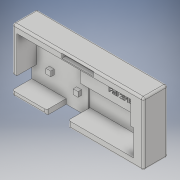
# Autodesk Inventor part: case3
Saved by Autodesk Inventor 2017 (Build 210142000, 142)
## iProperties
Created: 2016-12-02
Part Number: case3
Material: Generic
Document SubType Name: Modeling
Designer: SDL
Density: 1 g/cm^3
Appearance: Default
Author: SDL
Autodesk Inventor part; units mm, degrees
ref_plane "YZ Plane" through (0, 0, 0) normal (1, 0, 0) x (0, 1, 0)
ref_plane "XZ Plane" through (0, 0, 0) normal (0, 1, 0) x (-1, 0, 0)
ref_plane "XY Plane" through (0, 0, 0) normal (0, 0, 1) x (1, 0, 0)
sketch "Sketch1" plane through (0, 0, 0) normal (0, 0, 1) x (1, 0, 0)
  line L0 (0, 0) -> (133, 0)
  line L1 (133, 0) -> (133, 64)
  line L2 (133, 64) -> (0, 64)
  line L3 (0, 64) -> (0, 0)
  dimension "d0" = 133
  dimension "d1" = 64
  constraints: 8 end point, 2 parallel, 1 horizontal, 1 perpendicular
  measures "d0" distance of L2.end L1.end
  measures "d1" distance of L1.end L0.end
extrude "Extrusion1" add sketch "Sketch1" along normal blind 25
sketch "Sketch2" plane through (0, 0, 25) normal (0, 0, 1) x (1, 0, 0)
  line L0 (5, 5) -> (57, 5)
  line L1 (57, 5) -> (57, 57)
  line L2 (57, 57) -> (5, 57)
  line L3 (5, 57) -> (5, 5)
  dimension "d10" = 52
  dimension "d11" = 52
  constraints: 8 end point, 2 parallel, 1 horizontal, 1 perpendicular
  measures "d10" distance of L2.end L1.end
  measures "d11" distance of L1.end L0.end
extrude "Extrusion2" cut sketch "Sketch2" against normal blind 20
sketch "Sketch3" plane through (0, 0, 25) normal (0, 0, 1) x (1, 0, 0)
  line L0 (57, 57) -> (57, 5) projected
  line L1 (57, 7) -> (123, 7)
  line L2 (123, 7) -> (123, 33.5)
  line L3 (123, 33.5) -> (57, 33.5)
  line L4 (57, 33.5) -> (57, 7)
  point P0 (0, 0)
  dimension "d15" = 66
  dimension "d16" = 26.5
  constraints: 8 end point, 2 parallel, 1 horizontal, 1 perpendicular, 1 point on line
  measures "d15" distance of L3.end L2.end
  measures "d16" distance of L2.end L1.end
extrude "Extrusion3" cut sketch "Sketch3" against normal blind 22
sketch "Sketch4" plane through (0, 0, 3) normal (0, 0, 1) x (1, 0, 0)
  line L0 (123, 7) -> (57, 7) projected
  line L1 (57, 33.5) -> (123, 33.5) projected
  line L2 (123, 7) -> (110, 7)
  line L3 (110, 7) -> (110, 33.5)
  line L4 (110, 33.5) -> (123, 33.5)
  line L5 (123, 33.5) -> (123, 7)
  point P0 (0, 0)
  dimension "d19" = 13
  constraints: 8 end point, 2 parallel, 1 horizontal, 1 perpendicular, 1 point on line
  measures "d19" distance of L3.end L4.end
extrude "Extrusion4" cut sketch "Sketch4" against normal blind 25
sketch "Sketch5" plane through (0, 0, 25) normal (0, 0, 1) x (1, 0, 0)
  line L0 (57, 33.5) -> (110, 33.5) projected
  line L1 (57, 33.5) -> (120, 33.5)
  line L2 (120, 33.5) -> (120, 57)
  line L3 (120, 57) -> (57, 57)
  line L4 (57, 57) -> (57, 33.5)
  point P0 (0, 0)
  dimension "d22" = 63
  constraints: 8 end point, 2 parallel, 1 horizontal, 1 perpendicular
  measures "d22" distance of L3.end L2.end
extrude "Extrusion5" cut sketch "Sketch5" against normal blind 12
sketch "Sketch6" plane through (0, 0, 5) normal (0, 0, 1) x (1, 0, 0)
  line L0 (5.5, 56.5) -> (56, 5.5) construction
  line L1 (56, 55.5) -> (6, 5.5) construction
  line L2 (5.5, 56.5) -> (5.5, 53.5)
  line L3 (5.5, 53.5) -> (9.9, 53.5)
  line L4 (6, 5.5) -> (6, 22.2)
  line L5 (6, 22.2) -> (20.3, 22.2)
  line L6 (56, 5.5) -> (56, 18)
  line L7 (56, 18) -> (47.9, 18)
  line L8 (7.4, 56) -> (12.4, 56)
  line L9 (12.4, 56) -> (12.4, 51)
  line L10 (12.4, 51) -> (7.4, 51)
  line L11 (7.4, 51) -> (7.4, 56)
  line L12 (7.4, 56) -> (12.4, 51) construction
  line L13 (12.4, 56) -> (7.4, 51) construction
  line L14 (17.8, 24.7) -> (22.8, 24.7)
  line L15 (22.8, 24.7) -> (22.8, 19.7)
  line L16 (22.8, 19.7) -> (17.8, 19.7)
  line L17 (17.8, 19.7) -> (17.8, 24.7)
  line L18 (17.8, 24.7) -> (22.8, 19.7) construction
  line L19 (22.8, 24.7) -> (17.8, 19.7) construction
  line L20 (45.4, 20.5) -> (50.4, 20.5)
  line L21 (50.4, 20.5) -> (50.4, 15.5)
  line L22 (50.4, 15.5) -> (45.4, 15.5)
  line L23 (45.4, 15.5) -> (45.4, 20.5)
  line L24 (45.4, 20.5) -> (50.4, 15.5) construction
  line L25 (50.4, 20.5) -> (45.4, 15.5) construction
  point P0 (0, 0)
  point P1 (31.1232, 30.6232)
  dimension "d25" = 50
  dimension "d26" = 50
  dimension "d27" = 3
  dimension "d28" = 4.4
  dimension "d29" = 16.7
  dimension "d30" = 14.3
  dimension "d31" = 12.5
  dimension "d32" = 8.1
  dimension "d33" = 5
  dimension "d34" = 5
  dimension "d35" = 5
  dimension "d36" = 5
  dimension "d37" = 5
  dimension "d38" = 5
  constraints: 52 end point, 6 midpoint, 6 parallel, 6 perpendicular, 3 horizontal, 2 point on line
  measures "d25" distance of L0.end L1.end
  measures "d26" distance of L1.start L0.end
  measures "d27" distance of L0.start L2.end
  measures "d28" distance of L2.end L3.end
  measures "d29" distance of L1.end L4.end
  measures "d30" distance of L4.end L5.end
  measures "d31" distance of L0.end L6.end
  measures "d32" distance of L6.end L7.end
  measures "d33" distance of L9.end L10.end
  measures "d34" distance of L8.end L9.end
  measures "d35" distance of L15.end L16.end
  measures "d36" distance of L14.end L15.end
  measures "d37" distance of L21.end L22.end
  measures "d38" distance of L20.end L21.end
extrude "Extrusion6" add sketch "Sketch6" along normal blind 3.5
sketch "Sketch7" plane through (0, 0, 25) normal (0, 0, 1) x (1, 0, 0)
  line L0 (57, 0) -> (35, 0)
  line L1 (35, 0) -> (35, 5)
  line L2 (35, 5) -> (57, 5)
  line L3 (57, 5) -> (57, 0)
  line L4 (5, 5) -> (5, 57) projected
  line L5 (0, 64) -> (0, 0) projected
  line L6 (5, 5) -> (0, 5)
  line L7 (0, 5) -> (0, 20)
  line L8 (0, 20) -> (5, 20)
  line L9 (5, 20) -> (5, 5)
  dimension "d41" = 22
  dimension "d42" = 15
  constraints: 16 end point, 4 parallel, 2 horizontal, 2 perpendicular, 1 point on line
  measures "d41" distance of L1.end L2.end
  measures "d42" distance of L6.end L7.end
extrude "Extrusion7" cut sketch "Sketch7" against normal blind 20
sketch "Sketch8" plane through (0, 0, 25) normal (0, 0, 1) x (1, 0, 0)
  line L0 (0, 64) -> (0, 20) projected
  line L1 (133, 64) -> (0, 64) projected
  line L2 (82.5, 58) -> (50.5, 58)
  line L3 (50.5, 58) -> (50.5, 62.5)
  line L4 (50.5, 62.5) -> (82.5, 62.5)
  line L5 (82.5, 62.5) -> (82.5, 58)
  point P0 (0, 0)
  dimension "d49" = 32
  constraints: 8 end point, 2 parallel, 1 horizontal, 1 perpendicular
  measures "d49" distance of L3.end L4.end
extrude "Extrusion8" cut sketch "Sketch8" against normal blind 4
sketch "Sketch9" plane through (0, 0, 13) normal (0, 0, 1) x (1, 0, 0)
  line L0 (65.4851, 51.0922) -> (87.1486, 51.0922) construction
  line L1 (87.1486, 51.0922) -> (87.1486, 46.3193) construction
  line L2 (87.1486, 46.3193) -> (65.4851, 46.3193) construction
  line L3 (65.4851, 46.3193) -> (65.4851, 51.0922) construction
  line L4 (87.1486, 46.3193) -> (111.9776, 46.3193) construction
  line L5 (111.9776, 46.3193) -> (111.9776, 41.4723) construction
  line L6 (111.9776, 41.4723) -> (87.1486, 41.4723) construction
  line L7 (87.1486, 41.4723) -> (87.1486, 46.3193) construction
  line L8 (65.9493, 46.8186) -> (65.9493, 51.0186)
  line L9 (65.9493, 51.0186) -> (68.9905, 51.0186)
  line L10 (68.9905, 51.0186) -> (68.9905, 50.5224)
  line L11 (68.9905, 50.5224) -> (66.5063, 50.5224)
  line L12 (66.5063, 50.5224) -> (66.5063, 49.2387)
  line L13 (66.5063, 49.2387) -> (68.8336, 49.2387)
  line L14 (68.8336, 49.2387) -> (68.8336, 48.7425)
  line L15 (68.8336, 48.7425) -> (66.5063, 48.7425)
  line L16 (66.5063, 48.7425) -> (66.5063, 47.3148)
  line L17 (66.5063, 47.3148) -> (69.0865, 47.3148)
  line L18 (69.0865, 47.3148) -> (69.0865, 46.8186)
  line L19 (69.0865, 46.8186) -> (65.9493, 46.8186)
  line L20 (69.6627, 48.1695) -> (70.1877, 48.2143)
  spline S0 degree 2 poles (70.1877, 48.2143) (70.2261, 47.8974) (70.4982, 47.4941) (71.0712, 47.2444) (71.4298, 47.2444) knots 0 0 0 1 2 3 3 3
  spline S1 degree 2 poles (71.4298, 47.2444) (71.7467, 47.2444) (72.2365, 47.4332) (72.4734, 47.763) (72.4734, 47.9582) knots 0 0 0 1 2 3 3 3
  spline S2 degree 2 poles (72.4734, 47.9582) (72.4734, 48.1567) (72.2461, 48.4512) (71.9804, 48.5505) knots 0 0 0 1 2 2 2
  spline S3 degree 2 poles (71.9804, 48.5505) (71.8107, 48.6177) (70.6487, 48.8962) (70.415, 49.0211) knots 0 0 0 1 2 2 2
  spline S4 degree 2 poles (70.415, 49.0211) (70.1141, 49.1779) (69.8196, 49.6453) (69.8196, 49.9334) knots 0 0 0 1 2 2 2
  spline S5 degree 2 poles (69.8196, 49.9334) (69.8196, 50.2535) (70.1813, 50.8041) (70.876, 51.0922) (71.3017, 51.0922) knots 0 0 0 1 2 3 3 3
  spline S6 degree 2 poles (71.3017, 51.0922) (71.7691, 51.0922) (72.483, 50.7913) (72.8703, 50.2055) (72.8831, 49.8374) knots 0 0 0 1 2 3 3 3
  line L21 (72.8831, 49.8374) -> (72.3517, 49.7957)
  spline S7 degree 2 poles (72.3517, 49.7957) (72.3101, 50.1959) (71.8107, 50.6025) (71.3241, 50.6025) knots 0 0 0 1 2 2 2
  spline S8 degree 2 poles (71.3241, 50.6025) (70.8184, 50.6025) (70.3542, 50.2311) (70.3542, 49.9718) knots 0 0 0 1 2 2 2
  spline S9 degree 2 poles (70.3542, 49.9718) (70.3542, 49.7445) (70.5174, 49.5973) knots 0 0 0 1 1 1
  spline S10 degree 2 poles (70.5174, 49.5973) (70.6807, 49.4532) (72.0412, 49.1459) (72.2941, 49.0307) knots 0 0 0 1 2 2 2
  spline S11 degree 2 poles (72.2941, 49.0307) (72.6591, 48.861) (73.008, 48.3424) (73.008, 48.0063) knots 0 0 0 1 2 2 2
  spline S12 degree 2 poles (73.008, 48.0063) (73.008, 47.6701) (72.6238, 47.0779) (71.9036, 46.7482) (71.4554, 46.7482) knots 0 0 0 1 2 3 3 3
  spline S13 degree 2 poles (71.4554, 46.7482) (70.8824, 46.7482) (70.1141, 47.0811) (69.6755, 47.747) (69.6627, 48.1695) knots 0 0 0 1 2 3 3 3
  line L22 (73.7795, 46.8186) -> (73.7795, 51.0186)
  line L23 (73.7795, 51.0186) -> (76.8206, 51.0186)
  line L24 (76.8206, 51.0186) -> (76.8206, 50.5224)
  line L25 (76.8206, 50.5224) -> (74.3365, 50.5224)
  line L26 (74.3365, 50.5224) -> (74.3365, 49.2387)
  line L27 (74.3365, 49.2387) -> (76.6638, 49.2387)
  line L28 (76.6638, 49.2387) -> (76.6638, 48.7425)
  line L29 (76.6638, 48.7425) -> (74.3365, 48.7425)
  line L30 (74.3365, 48.7425) -> (74.3365, 47.3148)
  line L31 (74.3365, 47.3148) -> (76.9167, 47.3148)
  line L32 (76.9167, 47.3148) -> (76.9167, 46.8186)
  line L33 (76.9167, 46.8186) -> (73.7795, 46.8186)
  line L34 (77.4769, 47.9326) -> (77.9923, 47.9999)
  spline S14 degree 2 poles (77.9923, 47.9999) (78.0819, 47.5613) (78.5077, 47.1739) (78.815, 47.1739) knots 0 0 0 1 2 2 2
  spline S15 degree 2 poles (78.815, 47.1739) (79.1799, 47.1739) (79.6793, 47.6797) (79.6793, 48.0511) knots 0 0 0 1 2 2 2
  spline S16 degree 2 poles (79.6793, 48.0511) (79.6793, 48.4064) (79.2151, 48.8674) (78.8566, 48.8674) knots 0 0 0 1 2 2 2
  spline S17 degree 2 poles (78.8566, 48.8674) (78.7126, 48.8674) (78.4949, 48.8098) knots 0 0 0 1 1 1
  line L35 (78.4949, 48.8098) -> (78.5493, 49.2611)
  spline S18 degree 2 poles (78.5493, 49.2611) (78.6037, 49.2547) (78.6325, 49.2547) knots 0 0 0 1 1 1
  spline S19 degree 2 poles (78.6325, 49.2547) (78.9623, 49.2547) (79.4905, 49.6005) (79.4905, 49.9558) knots 0 0 0 1 2 2 2
  spline S20 degree 2 poles (79.4905, 49.9558) (79.4905, 50.2407) (79.1063, 50.6121) (78.8022, 50.6121) knots 0 0 0 1 2 2 2
  spline S21 degree 2 poles (78.8022, 50.6121) (78.5013, 50.6121) (78.1011, 50.2343) (78.0435, 49.8534) knots 0 0 0 1 2 2 2
  line L36 (78.0435, 49.8534) -> (77.5281, 49.9462)
  spline S22 degree 2 poles (77.5281, 49.9462) (77.6241, 50.4648) (78.2932, 51.0346) (78.7926, 51.0346) knots 0 0 0 1 2 2 2
  spline S23 degree 2 poles (78.7926, 51.0346) (79.1351, 51.0346) (79.7145, 50.7401) (80.0219, 50.2311) (80.0219, 49.9462) knots 0 0 0 1 2 3 3 3
  spline S24 degree 2 poles (80.0219, 49.9462) (80.0219, 49.6741) (79.7305, 49.2259) (79.4424, 49.0947) knots 0 0 0 1 2 2 2
  spline S25 degree 2 poles (79.4424, 49.0947) (79.817, 49.0082) (80.2267, 48.4672) (80.2267, 48.0607) knots 0 0 0 1 2 2 2
  spline S26 degree 2 poles (80.2267, 48.0607) (80.2267, 47.5133) (79.4232, 46.7482) (78.8118, 46.7482) knots 0 0 0 1 2 2 2
  spline S27 degree 2 poles (78.8118, 46.7482) (78.258, 46.7482) (77.5281, 47.4076) (77.4769, 47.9326) knots 0 0 0 1 2 2 2
  line L37 (83.444, 47.3148) -> (83.444, 46.8186)
  line L38 (83.444, 46.8186) -> (80.6685, 46.8186)
  spline S28 degree 2 poles (80.6685, 46.8186) (80.6621, 47.0043) (80.7293, 47.1772) knots 0 0 0 1 1 1
  spline S29 degree 2 poles (80.7293, 47.1772) (80.835, 47.4621) (81.3023, 48.0095) (81.7441, 48.3712) knots 0 0 0 1 2 2 2
  spline S30 degree 2 poles (81.7441, 48.3712) (82.426, 48.9346) (82.9062, 49.5877) (82.9062, 49.8822) knots 0 0 0 1 2 2 2
  spline S31 degree 2 poles (82.9062, 49.8822) (82.9062, 50.1895) (82.4676, 50.6089) (82.1155, 50.6089) knots 0 0 0 1 2 2 2
  spline S32 degree 2 poles (82.1155, 50.6089) (81.7441, 50.6089) (81.2991, 50.1607) (81.2959, 49.7669) knots 0 0 0 1 2 2 2
  line L39 (81.2959, 49.7669) -> (80.7645, 49.8214)
  spline S33 degree 2 poles (80.7645, 49.8214) (80.819, 50.4136) (81.5296, 51.0346) (82.1283, 51.0346) knots 0 0 0 1 2 2 2
  spline S34 degree 2 poles (82.1283, 51.0346) (82.7333, 51.0346) (83.4376, 50.3656) (83.4376, 49.8694) knots 0 0 0 1 2 2 2
  spline S35 degree 2 poles (83.4376, 49.8694) (83.4376, 49.6165) (83.2327, 49.1299) (82.7525, 48.5921) (82.1987, 48.1215) knots 0 0 0 1 2 3 3 3
  spline S36 degree 2 poles (82.1987, 48.1215) (81.7345, 47.7342) (81.472, 47.4557) (81.3856, 47.3148) knots 0 0 0 1 2 2 2
  line L40 (81.3856, 47.3148) -> (83.444, 47.3148)
  line L41 (84.001, 47.9326) -> (84.5164, 47.9999)
  spline S37 degree 2 poles (84.5164, 47.9999) (84.606, 47.5613) (85.0318, 47.1739) (85.3391, 47.1739) knots 0 0 0 1 2 2 2
  spline S38 degree 2 poles (85.3391, 47.1739) (85.704, 47.1739) (86.2034, 47.6797) (86.2034, 48.0511) knots 0 0 0 1 2 2 2
  spline S39 degree 2 poles (86.2034, 48.0511) (86.2034, 48.4064) (85.7392, 48.8674) (85.3807, 48.8674) knots 0 0 0 1 2 2 2
  spline S40 degree 2 poles (85.3807, 48.8674) (85.2366, 48.8674) (85.019, 48.8098) knots 0 0 0 1 1 1
  line L42 (85.019, 48.8098) -> (85.0734, 49.2611)
  spline S41 degree 2 poles (85.0734, 49.2611) (85.1278, 49.2547) (85.1566, 49.2547) knots 0 0 0 1 1 1
  spline S42 degree 2 poles (85.1566, 49.2547) (85.4863, 49.2547) (86.0145, 49.6005) (86.0145, 49.9558) knots 0 0 0 1 2 2 2
  spline S43 degree 2 poles (86.0145, 49.9558) (86.0145, 50.2407) (85.6304, 50.6121) (85.3263, 50.6121) knots 0 0 0 1 2 2 2
  spline S44 degree 2 poles (85.3263, 50.6121) (85.0254, 50.6121) (84.6252, 50.2343) (84.5676, 49.8534) knots 0 0 0 1 2 2 2
  line L43 (84.5676, 49.8534) -> (84.0522, 49.9462)
  spline S45 degree 2 poles (84.0522, 49.9462) (84.1482, 50.4648) (84.8173, 51.0346) (85.3167, 51.0346) knots 0 0 0 1 2 2 2
  spline S46 degree 2 poles (85.3167, 51.0346) (85.6592, 51.0346) (86.2386, 50.7401) (86.5459, 50.2311) (86.5459, 49.9462) knots 0 0 0 1 2 3 3 3
  spline S47 degree 2 poles (86.5459, 49.9462) (86.5459, 49.6741) (86.2546, 49.2259) (85.9665, 49.0947) knots 0 0 0 1 2 2 2
  spline S48 degree 2 poles (85.9665, 49.0947) (86.3411, 49.0082) (86.7508, 48.4672) (86.7508, 48.0607) knots 0 0 0 1 2 2 2
  spline S49 degree 2 poles (86.7508, 48.0607) (86.7508, 47.5133) (85.9473, 46.7482) (85.3359, 46.7482) knots 0 0 0 1 2 2 2
  spline S50 degree 2 poles (85.3359, 46.7482) (84.7821, 46.7482) (84.0522, 47.4076) (84.001, 47.9326) knots 0 0 0 1 2 2 2
  line L44 (87.6288, 42.1033) -> (87.6288, 46.3033)
  line L45 (87.6288, 46.3033) -> (90.4651, 46.3033)
  line L46 (90.4651, 46.3033) -> (90.4651, 45.8072)
  line L47 (90.4651, 45.8072) -> (88.1858, 45.8072)
  line L48 (88.1858, 45.8072) -> (88.1858, 44.5075)
  line L49 (88.1858, 44.5075) -> (90.1578, 44.5075)
  line L50 (90.1578, 44.5075) -> (90.1578, 44.0113)
  line L51 (90.1578, 44.0113) -> (88.1858, 44.0113)
  line L52 (88.1858, 44.0113) -> (88.1858, 42.1033)
  line L53 (88.1858, 42.1033) -> (87.6288, 42.1033)
  spline S51 degree 2 poles (93.1061, 42.4779) (92.818, 42.2346) (92.2898, 42.0361) (91.9857, 42.0361) knots 0 0 0 1 2 2 2
  spline S52 degree 2 poles (91.9857, 42.0361) (91.4831, 42.0361) (90.9453, 42.5259) (90.9453, 42.9068) knots 0 0 0 1 2 2 2
  spline S53 degree 2 poles (90.9453, 42.9068) (90.9453, 43.1309) (91.1502, 43.4991) (91.4767, 43.7232) (91.6848, 43.7776) knots 0 0 0 1 2 3 3 3
  spline S54 degree 2 poles (91.6848, 43.7776) (91.8352, 43.8192) (92.1425, 43.8576) knots 0 0 0 1 1 1
  spline S55 degree 2 poles (92.1425, 43.8576) (92.7668, 43.9312) (93.0613, 44.0337) knots 0 0 0 1 1 1
  spline S56 degree 2 poles (93.0613, 44.0337) (93.0645, 44.1393) (93.0645, 44.1681) knots 0 0 0 1 1 1
  spline S57 degree 2 poles (93.0645, 44.1681) (93.0645, 44.485) (92.9172, 44.6131) knots 0 0 0 1 1 1
  spline S58 degree 2 poles (92.9172, 44.6131) (92.7219, 44.7892) (92.3314, 44.7892) knots 0 0 0 1 1 1
  spline S59 degree 2 poles (92.3314, 44.7892) (91.9697, 44.7892) (91.6239, 44.5331) (91.5407, 44.2097) knots 0 0 0 1 2 2 2
  line L54 (91.5407, 44.2097) -> (91.0349, 44.277)
  spline S60 degree 2 poles (91.0349, 44.277) (91.1021, 44.6003) (91.4191, 45.0004) (92.0145, 45.2149) (92.405, 45.2149) knots 0 0 0 1 2 3 3 3
  spline S61 degree 2 poles (92.405, 45.2149) (92.7956, 45.2149) (93.2822, 45.0325) (93.5127, 44.7539) (93.5575, 44.5427) knots 0 0 0 1 2 3 3 3
  spline S62 degree 2 poles (93.5575, 44.5427) (93.5831, 44.4082) (93.5831, 44.0657) knots 0 0 0 1 1 1
  line L55 (93.5831, 44.0657) -> (93.5831, 43.3774)
  spline S63 degree 2 poles (93.5831, 43.3774) (93.5831, 42.6604) (93.6503, 42.2794) (93.7463, 42.1033) knots 0 0 0 1 2 2 2
  line L56 (93.7463, 42.1033) -> (93.2085, 42.1033)
  spline S64 degree 2 poles (93.2085, 42.1033) (93.1285, 42.2634) (93.1061, 42.4779) knots 0 0 0 1 1 1
  spline S65 degree 2 poles (93.0645, 43.6303) (92.7828, 43.5151) (92.2226, 43.435) knots 0 0 0 1 1 1
  spline S66 degree 2 poles (92.2226, 43.435) (91.9024, 43.3902) (91.6399, 43.275) (91.4959, 43.0541) (91.4959, 42.9197) knots 0 0 0 1 2 3 3 3
  spline S67 degree 2 poles (91.4959, 42.9197) (91.4959, 42.7148) (91.8064, 42.4395) (92.1073, 42.4395) knots 0 0 0 1 2 2 2
  spline S68 degree 2 poles (92.1073, 42.4395) (92.405, 42.4395) (92.8692, 42.6988) (92.978, 42.9261) knots 0 0 0 1 2 2 2
  spline S69 degree 2 poles (92.978, 42.9261) (93.0613, 43.1021) (93.0613, 43.4415) knots 0 0 0 1 1 1
  line L57 (93.0613, 43.4415) -> (93.0645, 43.6303)
  line L58 (94.3706, 42.1033) -> (94.3706, 46.3033)
  line L59 (94.3706, 46.3033) -> (94.886, 46.3033)
  line L60 (94.886, 46.3033) -> (94.886, 42.1033)
  line L61 (94.886, 42.1033) -> (94.3706, 42.1033)
  line L62 (95.6735, 42.1033) -> (95.6735, 46.3033)
  line L63 (95.6735, 46.3033) -> (96.1889, 46.3033)
  line L64 (96.1889, 46.3033) -> (96.1889, 42.1033)
  line L65 (96.1889, 42.1033) -> (95.6735, 42.1033)
  line L66 (101.1828, 42.5995) -> (101.1828, 42.1033)
  line L67 (101.1828, 42.1033) -> (98.4073, 42.1033)
  spline S70 degree 2 poles (98.4073, 42.1033) (98.4009, 42.289) (98.4681, 42.4619) knots 0 0 0 1 1 1
  spline S71 degree 2 poles (98.4681, 42.4619) (98.5738, 42.7468) (99.0412, 43.2942) (99.4829, 43.6559) knots 0 0 0 1 2 2 2
  spline S72 degree 2 poles (99.4829, 43.6559) (100.1648, 44.2193) (100.645, 44.8724) (100.645, 45.1669) knots 0 0 0 1 2 2 2
  spline S73 degree 2 poles (100.645, 45.1669) (100.645, 45.4742) (100.2064, 45.8936) (99.8543, 45.8936) knots 0 0 0 1 2 2 2
  spline S74 degree 2 poles (99.8543, 45.8936) (99.4829, 45.8936) (99.038, 45.4454) (99.0348, 45.0517) knots 0 0 0 1 2 2 2
  line L68 (99.0348, 45.0517) -> (98.5034, 45.1061)
  spline S75 degree 2 poles (98.5034, 45.1061) (98.5578, 45.6983) (99.2684, 46.3193) (99.8671, 46.3193) knots 0 0 0 1 2 2 2
  spline S76 degree 2 poles (99.8671, 46.3193) (100.4721, 46.3193) (101.1764, 45.6503) (101.1764, 45.1541) knots 0 0 0 1 2 2 2
  spline S77 degree 2 poles (101.1764, 45.1541) (101.1764, 44.9012) (100.9715, 44.4146) (100.4913, 43.8768) (99.9375, 43.4062) knots 0 0 0 1 2 3 3 3
  spline S78 degree 2 poles (99.9375, 43.4062) (99.4733, 43.0189) (99.2108, 42.7404) (99.1244, 42.5995) knots 0 0 0 1 2 2 2
  line L69 (99.1244, 42.5995) -> (101.1828, 42.5995)
  spline S79 degree 2 poles (101.7366, 44.1745) (101.7366, 44.9204) (102.0439, 45.8296) (102.6457, 46.3193) (103.1067, 46.3193) knots 0 0 0 1 2 3 3 3
  spline S80 degree 2 poles (103.1067, 46.3193) (103.4428, 46.3193) (103.955, 46.0472) (104.2848, 45.535) (104.4736, 44.7988) (104.4736, 44.1745) knots 0 0 0 1 2 3 4 4 4
  spline S81 degree 2 poles (104.4736, 44.1745) (104.4736, 43.435) (104.1695, 42.5259) (103.5645, 42.0329) (103.1067, 42.0329) knots 0 0 0 1 2 3 3 3
  spline S82 degree 2 poles (103.1067, 42.0329) (102.4985, 42.0329) (102.1527, 42.4651) knots 0 0 0 1 1 1
  spline S83 degree 2 poles (102.1527, 42.4651) (101.7366, 42.9933) (101.7366, 44.1745) knots 0 0 0 1 1 1
  spline S84 degree 2 poles (102.268, 44.1745) (102.268, 43.1373) (102.7514, 42.4555) (103.1067, 42.4555) knots 0 0 0 1 2 2 2
  spline S85 degree 2 poles (103.1067, 42.4555) (103.4588, 42.4555) (103.9422, 43.1405) (103.9422, 44.1745) knots 0 0 0 1 2 2 2
  spline S86 degree 2 poles (103.9422, 44.1745) (103.9422, 45.2117) (103.4588, 45.8936) (103.1003, 45.8936) knots 0 0 0 1 2 2 2
  spline S87 degree 2 poles (103.1003, 45.8936) (102.745, 45.8936) (102.5337, 45.5927) knots 0 0 0 1 1 1
  spline S88 degree 2 poles (102.5337, 45.5927) (102.268, 45.2085) (102.268, 44.1745) knots 0 0 0 1 1 1
  line L70 (106.9386, 42.1033) -> (106.4232, 42.1033)
  line L71 (106.4232, 42.1033) -> (106.4232, 45.3878)
  spline S89 degree 2 poles (106.4232, 45.3878) (106.2375, 45.2117) (105.6325, 44.8564) (105.3924, 44.7668) knots 0 0 0 1 2 2 2
  line L72 (105.3924, 44.7668) -> (105.3924, 45.2661)
  spline S90 degree 2 poles (105.3924, 45.2661) (105.8245, 45.4678) (106.4712, 46.0472) (106.6056, 46.3193) knots 0 0 0 1 2 2 2
  line L73 (106.6056, 46.3193) -> (106.9386, 46.3193)
  line L74 (106.9386, 46.3193) -> (106.9386, 42.1033)
  line L75 (110.9401, 45.2725) -> (110.4279, 45.2309)
  spline S91 degree 2 poles (110.4279, 45.2309) (110.3575, 45.535) (110.2326, 45.6759) knots 0 0 0 1 1 1
  spline S92 degree 2 poles (110.2326, 45.6759) (110.0213, 45.8968) (109.714, 45.8968) knots 0 0 0 1 1 1
  spline S93 degree 2 poles (109.714, 45.8968) (109.4675, 45.8968) (109.2819, 45.7591) knots 0 0 0 1 1 1
  spline S94 degree 2 poles (109.2819, 45.7591) (109.0386, 45.5831) (108.7569, 44.898) (108.7505, 44.2674) knots 0 0 0 1 2 2 2
  spline S95 degree 2 poles (108.7505, 44.2674) (108.9361, 44.5523) (109.4771, 44.8276) (109.7716, 44.8276) knots 0 0 0 1 2 2 2
  spline S96 degree 2 poles (109.7716, 44.8276) (110.287, 44.8276) (111.0137, 44.0689) (111.0137, 43.4671) knots 0 0 0 1 2 2 2
  spline S97 degree 2 poles (111.0137, 43.4671) (111.0137, 43.0733) (110.6712, 42.3947) (110.0758, 42.0329) (109.698, 42.0329) knots 0 0 0 1 2 3 3 3
  spline S98 degree 2 poles (109.698, 42.0329) (109.0514, 42.0329) (108.2383, 42.9805) (108.2383, 44.0689) knots 0 0 0 1 2 2 2
  spline S99 degree 2 poles (108.2383, 44.0689) (108.2383, 45.2854) (108.6896, 45.8392) knots 0 0 0 1 1 1
  spline S100 degree 2 poles (108.6896, 45.8392) (109.0802, 46.3193) (109.746, 46.3193) knots 0 0 0 1 1 1
  spline S101 degree 2 poles (109.746, 46.3193) (110.2422, 46.3193) (110.8761, 45.7623) (110.9401, 45.2725) knots 0 0 0 1 2 2 2
  spline S102 degree 2 poles (108.8305, 43.4639) (108.8305, 43.1982) (109.0578, 42.7116) (109.4611, 42.4555) (109.6852, 42.4555) knots 0 0 0 1 2 3 3 3
  spline S103 degree 2 poles (109.6852, 42.4555) (110.0149, 42.4555) (110.4823, 42.9837) (110.4823, 43.435) knots 0 0 0 1 2 2 2
  spline S104 degree 2 poles (110.4823, 43.435) (110.4823, 43.8704) (110.0213, 44.373) (109.666, 44.373) knots 0 0 0 1 2 2 2
  spline S105 degree 2 poles (109.666, 44.373) (109.3171, 44.373) (108.8305, 43.8704) (108.8305, 43.4639) knots 0 0 0 1 2 2 2
  point P0 (0, 0)
  constraints: 1 coincident, 4 other
extrude "Extrusion9" add sketch "Sketch9" along normal blind 1.5
fillet "Fillet1" radius 2 8 edges at (66.5, 64, 25) (0, 42, 25) (0, 2.5, 25) (17.5, 0, 25) (35, 2.5, 25) (57, 3.5, 25) (95, 0, 25) (133, 32, 25)
fillet "Fillet3" radius 2 12 edges at (0.5858, 63.4142, 24.4142) (0, 64, 11.5) (0.5858, 0.5858, 24.4142) (0, 0, 11.5) (0, 32, 0) (66.5, 0, 0) (66.5, 64, 0) (132.4142, 63.4142, 24.4142) (133, 64, 11.5) (133, 32, 0) (132.4142, 0.5858, 24.4142) (133, 0, 11.5)
body "Solid1"
